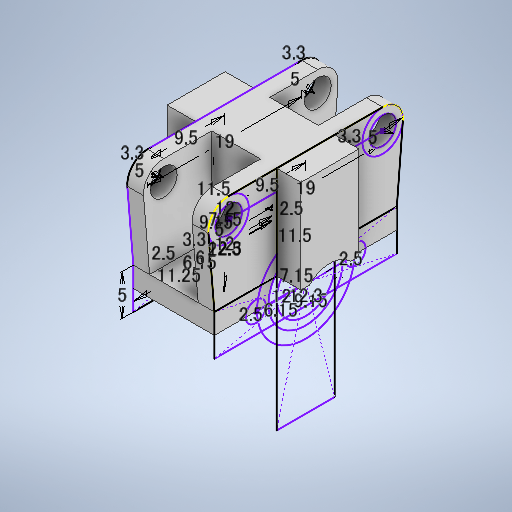
# Autodesk Inventor part: ikafly5.0c
Saved by Autodesk Inventor 2025 (Build 290162000, 162)
## iProperties
Created: 2024-06-20
Part Number: ikafly5.0c
Material: 一般
Document SubType Name: Modeling
Designer: Saigusa
Density: 1 g/cm^3
Appearance: 既定
Author: Saigusa
Autodesk Inventor part; units mm, degrees
ref_plane "YZ Plane" through (0, 0, 0) normal (1, 0, 0) x (0, 1, 0)
ref_plane "XZ Plane" through (0, 0, 0) normal (0, 1, 0) x (-1, 0, 0)
ref_plane "XY Plane" through (0, 0, 0) normal (0, 0, 1) x (1, 0, 0)
sketch "スケッチ1" plane through (0, 0, 0) normal (1, 0, 0) x (0, 1, 0)
  circle A0 centre (0, 0) radius 4.575
  circle A1 centre (0, 0) radius 3.575
  line L0 (0, 0) -> (0, 6)
  line L1 (0, 6) -> (0, -6)
  line L2 (0, 0) -> (11.5, 0)
  line L3 (11.5, 0) -> (11.5, 9.5)
  line L4 (11.5, 9.5) -> (11.5, -9.5)
  circle A2 centre (11.5, 9.5) radius 1.65
  circle A3 centre (11.5, -9.5) radius 1.65
  line L5 (0, 0) -> (0, 11.25)
  line L6 (0, 11.25) -> (0, -11.25)
  line L7 (-2.5, -11.25) -> (2.5, -11.25)
  line L8 (2.5, -11.25) -> (2.5, 11.25)
  line L9 (2.5, 11.25) -> (-2.5, 11.25)
  line L10 (-2.5, 11.25) -> (-2.5, -11.25)
  line L11 (-2.5, -11.25) -> (2.5, 11.25) construction
  line L12 (2.5, -11.25) -> (-2.5, 11.25) construction
  circle A4 centre (11.5, 9.5) radius 2.5
  circle A5 centre (11.5, -9.5) radius 2.5
  line L13 (2.5, 11.25) -> (11.2899, 11.9912)
  line L14 (2.5, -11.25) -> (11.2899, -11.9912)
  line L15 (14, 9.5) -> (14, -9.5)
  line L16 (0, -3.575) -> (14, -3.575)
  line L17 (0, 3.575) -> (14, 3.575)
  circle A6 centre (0, 0) radius 6
  line L18 (0, 0) -> (0, 6.15)
  line L19 (0, 6.15) -> (0, -6.15)
  circle A7 centre (0, 6.15) radius 1.25
  circle A8 centre (0, -6.15) radius 1.25
  point P0 (0, 4.575)
  point P1 (0, -4.575)
  point P2 (2.5, 3.575)
  point P3 (2.5, 2.5555)
  point P4 (2.5, -2.5555)
  point P5 (2.5, -3.575)
  point P6 (0, 7.4)
  point P7 (0, 4.9)
  point P8 (0, -4.9)
  point P9 (0, -7.4)
  point P10 (2.5, 5.4544)
  point P11 (2.5, -5.4544)
  point P12 (4.8186, 3.575)
  point P13 (4.8186, -3.575)
  point P14 (2.8548, 3.575)
  point P15 (2.8548, -3.575)
  dimension "d0" = 9.15
  dimension "d1" = 7.15
  dimension "d2" = 6
  dimension "d3" = 12
  dimension "d6" = 11.5
  dimension "d7" = 9.5
  dimension "d8" = 19
  dimension "d9" = 3.3
  dimension "d10" = 3.3
  dimension "d11" = 11.25
  dimension "d12" = 22.5
  dimension "d13" = 5
  dimension "d14" = 5
  dimension "d15" = 5
  dimension "d28" = 12
  dimension "d29" = 6.15
  dimension "d30" = 12.3
  dimension "d31" = 2.5
  dimension "d32" = 2.5
  constraints: 40 end point, 9 centre point, 9 coincident, 8 point on line, 6 point on circle, 5 tangent, 4 perpendicular, 2 horizontal, 2 midpoint, 2 parallel, 1 vertical
  measures "d0" diameter of A0
  measures "d1" diameter of A1
  measures "d2" distance of L0.start L0.end
  measures "d3" distance of L0.end L1.end
  measures "d6" distance of L0.start L2.end
  measures "d7" distance of L2.end L3.end
  measures "d8" distance of L3.end L4.end
  measures "d9" diameter of A2
  measures "d10" diameter of A3
  measures "d11" distance of L0.start L5.end
  measures "d12" distance of L5.end L6.end
  measures "d13" distance of L9.end L8.end
  measures "d14" diameter of A4
  measures "d15" diameter of A5
  measures "d28" diameter of A6
  measures "d29" distance of L18.start L18.end
  measures "d30" distance of L18.end L19.end
  measures "d31" diameter of A7
  measures "d32" diameter of A8
extrude "押し出し7" add sketch "スケッチ1" along normal blind 2 contours L2 A6 L16 A0 | A0 L17 A6 L2 | A0 L8 A6 L17 | L16 A6 L8 A0 | A6 L17 L3 L2 | L2 L4 L16 A6 | A0 L0 A7 A6 L8 | A6 L8 L13 A4 L3 L17 | L8 A6 A8 L1 A0 | L16 L4 A5 L14 L8 A6 | L3 L17 L15 L16 L4 | A6 A7 L5 L9 L8 | L3 A4 L15 L17 | L8 L7 L6 A8 A6 | L16 L15 A5 L4 | A4 | A5
extrude "押し出し8" add sketch "スケッチ1" along normal blind 10 contours L2 A6 L16 A0 | A0 L17 A6 L2 | A0 L8 A6 L17 | L16 A6 L8 A0 | A6 L17 L3 L2 | L2 L4 L16 A6 | A0 L0 A7 A6 L8 | L8 A6 A8 L1 A0 | L3 L17 L15 L16 L4 | A6 A7 L5 L9 L8 | L8 L7 L6 A8 A6 | L0 A6 A7 | A6 L5 A7 | A8 A6 L1 | A8 L6 A6 picked at (0.2292, 5.6392) picked at (0.3961, 6.4211) picked at (0.2292, -5.6392) picked at (0.3961, -6.4211)
sketch "スケッチ6" plane through (10, 0, 0) normal (1, 0, 0) x (0, 0, -1)
  line L0 (0, 0) -> (-6.15, 0)
  line L1 (-6.15, 0) -> (6.15, 0)
  circle A0 centre (-6.15, 0) radius 1.25
  circle A1 centre (6.15, 0) radius 1.25
  line L2 (-11.25, 2.5) -> (11.25, 2.5)
  line L3 (11.25, 2.5) -> (11.25, -2.5)
  line L4 (11.25, -2.5) -> (-11.25, -2.5)
  line L5 (-11.25, -2.5) -> (-11.25, 2.5)
  line L6 (-11.25, 2.5) -> (11.25, -2.5) construction
  line L7 (11.25, 2.5) -> (-11.25, -2.5) construction
  line L8 (0, 0) -> (0, 11.5)
  line L9 (0, 11.5) -> (-9.5, 11.5)
  line L10 (-9.5, 11.5) -> (9.5, 11.5)
  circle A2 centre (-9.5, 11.5) radius 1.65
  circle A3 centre (-9.5, 11.5) radius 2.5
  circle A4 centre (9.5, 11.5) radius 1.65
  circle A5 centre (9.5, 11.5) radius 2.5
  circle A6 centre (0, 0) radius 6
  circle A7 centre (0, 0) radius 4.575
  arc A8 (11.9912, 11.2899) -> (9.5, 14) centre (9.5, 11.5) ccw projected
  line L11 (11.25, 2.5) -> (11.9912, 11.2899)
  line L12 (-11.9912, 11.2899) -> (-11.25, 2.5) projected
  line L13 (-11.25, 2.5) -> (-11.9912, 11.2899)
  line L14 (9.5, 14) -> (-9.5, 14) projected
  arc A9 (-9.5, 14) -> (-11.9912, 11.2899) centre (-9.5, 11.5) ccw projected
  line L15 (-9.5, 14) -> (9.5, 14)
  circle A10 centre (0, 0) radius 3.575
  line L16 (-3.575, 14) -> (-3.575, 4.8186) projected
  line L17 (3.575, -14) -> (-3.575, -14)
  line L18 (-3.575, -14) -> (-3.575, 14)
  line L19 (-3.575, 14) -> (3.575, 14)
  line L20 (3.575, 14) -> (3.575, -14)
  line L21 (3.575, -14) -> (-3.575, 14) construction
  line L22 (-3.575, -14) -> (3.575, 14) construction
  point P0 (-5.4544, 2.5)
  point P1 (5.4544, 2.5)
  point P2 (7, 11.5)
  point P3 (-7, 11.5)
  point P4 (-3.575, 11.5)
  point P5 (-3.575, 4.8186)
  point P6 (-3.575, 2.5)
  point P7 (-2.5555, 2.5)
  point P8 (2.5555, 2.5)
  point P9 (3.575, 2.5)
  point P10 (3.575, 11.5)
  dimension "d69" = 12
  dimension "d56" = 6.15
  dimension "d57" = 12.3
  dimension "d58" = 2.5
  dimension "d59" = 2.5
  dimension "d62" = 11.5
  dimension "d63" = 9.5
  dimension "d64" = 19
  dimension "d65" = 3.3
  dimension "d66" = 5
  dimension "d67" = 3.3
  dimension "d68" = 5
  dimension "d70" = 9.15
  dimension "d79" = 7.15
  constraints: 40 end point, 9 coincident, 8 centre point, 5 equal length, 4 horizontal, 4 midpoint, 3 perpendicular, 2 point on line, 2 tangent, 1 vertical, 2 other
  measures "d56" distance of L0.start L0.end
  measures "d57" distance of L0.end L1.end
  measures "d58" diameter of A0
  measures "d59" diameter of A1
  measures "d62" distance of L0.start L8.end
  measures "d63" distance of L8.end L9.end
  measures "d64" distance of L9.end L10.end
  measures "d65" diameter of A2
  measures "d66" diameter of A3
  measures "d67" diameter of A4
  measures "d68" diameter of A5
  measures "d70" diameter of A7
  measures "d79" diameter of A10
extrude "押し出し9" add sketch "スケッチ6" against normal blind 2 contours L2 L12 A3 L9 L16 A6 | L16 L9 L8 A6 | A6 L20 L10 A5 L11 L2 | A6 L8 L10 L20 | L16 L14 L20 L10 L9 | L9 A3 L14 L16 | L20 L14 A5 L10 | A3 | A5
extrude "押し出し10" add sketch "スケッチ1" against normal blind 0.5 contours L2 A6 L16 A0 | A0 L17 A6 L2 | A6 L17 L3 L2 | L2 L4 L16 A6 | L3 L17 L15 L16 L4
sketch "スケッチ7" plane through (-0.5, 0, 0) normal (-1, 0, 0) x (0, 0, 1)
  circle A0 centre (0, 0) radius 3.575
  line L0 (-9.5, 14) -> (9.5, 14) projected
  line L1 (-3.575, 14) -> (3.575, 14)
  circle A1 centre (0, 0) radius 4.575
  line L2 (-11.25, 0) -> (-11.25, 2.5) projected
  line L3 (11.25, -2.5) -> (-11.25, -2.5)
  line L4 (-11.25, -2.5) -> (-11.25, 2.5)
  line L5 (-11.25, 2.5) -> (11.25, 2.5)
  line L6 (11.25, 2.5) -> (11.25, -2.5)
  line L7 (11.25, -2.5) -> (-11.25, 2.5) construction
  line L8 (-11.25, -2.5) -> (11.25, 2.5) construction
  line L9 (-3.575, 14) -> (-3.575, 0)
  line L10 (3.575, 14) -> (3.575, 0)
  point P0 (-3.575, 2.5)
  point P1 (-2.5555, 2.5)
  point P2 (2.5555, 2.5)
  point P3 (3.575, 2.5)
  dimension "d75" = 7.15
  dimension "d76" = 5
  constraints: 18 end point, 2 centre point, 2 coincident, 2 midpoint, 2 parallel, 2 point on circle, 2 point on line, 2 tangent, 1 horizontal, 1 perpendicular
  measures "d75" diameter of A0
  measures "d76" distance of L3.end L2.end
extrude "押し出し11" add sketch "スケッチ7" along normal blind 3 contours A0 L5 L9 A1 L10 | A1 L9 L0 L10
extrude "押し出し12" add sketch "スケッチ6" along normal blind 3 contours L2 L18 A7 L8 A10 | A10 L8 A7 L20 L2 | L18 A6 L8 A7 | A7 L8 A6 L20 | L16 L9 L8 A6 | A6 L8 L10 L20 | L16 L14 L20 L10 L9
hole "穴1" at (0, 0, -6.15) at (0, 0, 6.15) direction (1, 0, 0) diameter 2.4 depth 3
